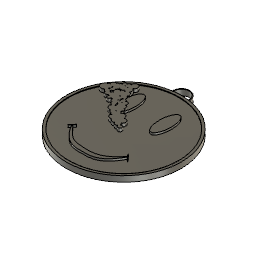
Comedian_Badge_v.2 (Autodesk Fusion 360 design; units mm, degrees)
part number: 2026-01-01-18-05-26-617
part number: 2026-01-01-18-09-21-540
part number: 2026-01-01-18-09-43-519
part number: 2026-01-01-18-09-54-607
Autodesk Fusion 360 part; units mm, degrees
sketch "Base" plane through (0, 0, 0) normal (0, 0, 1) x (1, 0, 0) in component "Base"
  circle A0 centre (0, 0) radius 32.5
  circle A1 centre (0, 0) radius 34
  arc A2 (4.9865, 33.6324) -> (-4.9865, 33.6324) centre (0, 34) ccw
  arc A3 (4.4878, 33.6691) -> (-4.4878, 33.6691) centre (0, 34) ccw
  dimension "d1" = 65
  dimension "d2" = 1.5
  dimension "d7" = 10
  dimension "d8" = -0.5
  constraint coincident A0.centre A1.centre
  constraint coincident A1 A2.centre
  constraint vertical A0.centre A2.centre
  constraint coincident A1 A2.start
  constraint coincident A1 A2.end
  measures "d1" diameter of A0
  measures "d7" diameter of A2
extrude "Face" add sketch "Base" along normal blind 3 contours A0 makes body 1 in component "Base"
extrude "Boundary" add sketch "Base" along normal blind 3.4 contours A1 bodies 1 in component "Base"
extrude "Extrude3" add sketch "Base" along normal blind 3.4 contours A1 A2 A3 bodies 1 in component "Base"
sketch "Face" plane through (0, 0, 3) normal (0, 0, 1) x (-1, 0, 0) in component "Eyes, Mouth"
  circle A0 centre (0, 0) radius 32.5
  line L0 (0, -32.5) -> (0, 32.5) construction
  line L1 (32.5, 0) -> (-32.5, 0) construction
  line L2 (32.5, 0) -> (0, 0) construction
  line L3 (16.25, 0) -> (16.25, -28.1458) construction
  line L4 (0, 0) -> (-32.5, 0) construction
  line L5 (0, 0) -> (-32.5, 0) construction
  line L6 (-16.25, 0) -> (-16.25, -28.1458) construction
  line L7 (16.25, 0) -> (16.25, 28.1458) construction
  line L8 (-16.25, 0) -> (-16.25, 28.1458) construction
  line L9 (10.514, -30.7523) -> (10.5048, 0) construction
  line L10 (-10.51, 0) -> (-10.51, -30.7537) construction
  line L11 (29.33, -14) -> (-29.33, -14) construction
  ellipse E0 centre (10.509, -14) end of major axis (10.5116, -22.6) minor radius 3.5
  line L12 (10.5064, -5.4) -> (10.5116, -22.6) construction
  line L13 (7.009, -14.001) -> (14.009, -13.999) construction
  ellipse E1 centre (-10.53, -14) end of major axis (-10.5274, -22.6) minor radius 3.5
  line L14 (15.0904, 12.7622) -> (17.4096, 15.3836)
  line L15 (16.25, 14.0729) -> (-16.25, 14.0729) construction
  line L16 (-15.0938, 12.7592) -> (-17.4062, 15.3866)
  spline S0 degree 5 poles (16.25, 14.0729) (16.3, 14.0848) (16.3341, 14.1993) (16.1818, 14.6464) (15.5759, 15.7501) (14.2531, 17.6838) (12.5268, 19.7926) (10.5746, 21.7057) (8.5494, 23.1547) (6.5388, 24.0726) (4.5785, 24.5327) (2.6673, 24.6856) (0.7818, 24.6946) (-1.1097, 24.6783) (-3.031, 24.6326) (-4.9909, 24.4416) (-6.9805, 23.9504) (-8.9701, 23.0199) (-10.9061, 21.5858) (-12.7062, 19.7261) (-14.2606, 17.6936) (-15.454, 15.8206) (-16.1842, 14.4433) (-16.3813, 13.8224) (-16.0298, 14.0561) (-15.1804, 15.0207) (-13.9095, 16.4685) (-12.276, 18.1183) (-10.3075, 19.7152) (-8.0314, 21.0469) (-5.4863, 21.9624) (-2.7594, 22.4114) (0.0273, 22.4249) (2.6134, 22.2412) (4.8105, 22.0395) (6.6671, 21.7352) (8.3079, 21.1812) (9.891, 20.2249) (11.5227, 18.8139) (13.1704, 17.1114) (14.6738, 15.4616) (15.5937, 14.498) (16.0342, 14.1281) (16.2, 14.0611) (16.25, 14.0729) knots 0 0 0 0 0 0 0.025 0.05 0.075 0.1 0.125 0.15 0.175 0.2 0.225 0.25 0.275 0.3 0.325 0.35 0.375 0.4 0.425 0.45 0.475 0.5 0.525 0.55 0.575 0.6 0.625 0.65 0.675 0.7 0.725 0.75 0.775 0.8 0.825 0.85 0.875 0.9 0.925 0.95 0.975 1 1 1 1 1 1
  line L17 (-4.0312, 22.4795) -> (4.0312, 22.2695)
  line L18 (15.3272, 12.5528) -> (17.6464, 15.1741)
  spline S1 degree 5 poles (17.6464, 15.1741) (17.6631, 15.193) (17.6879, 15.2308) (17.6992, 15.2873) (17.6702, 15.3599) (17.5911, 15.4298) (17.5155, 15.4498) (17.4608, 15.4318) (17.4263, 15.4025) (17.4096, 15.3836) knots 0 0 0 0 0 0 0.2 0.4 0.6 0.8 1 1 1 1 1 1
  spline S2 degree 5 poles (15.3272, 12.5528) (15.3104, 12.5338) (15.276, 12.5046) (15.2212, 12.4866) (15.1457, 12.5065) (15.0666, 12.5765) (15.0376, 12.649) (15.0488, 12.7055) (15.0737, 12.7433) (15.0904, 12.7622) knots 0 0 0 0 0 0 0.2 0.4 0.6 0.8 1 1 1 1 1 1
  line L19 (-15.3311, 12.5505) -> (-17.6434, 15.1778)
  spline S3 degree 5 poles (-15.3311, 12.5505) (-15.3144, 12.5315) (-15.28, 12.5022) (-15.2253, 12.484) (-15.1498, 12.5037) (-15.0705, 12.5735) (-15.0414, 12.6459) (-15.0524, 12.7024) (-15.0771, 12.7403) (-15.0938, 12.7592) knots 0 0 0 0 0 0 0.2 0.4 0.6 0.8 1 1 1 1 1 1
  spline S4 degree 5 poles (-17.4062, 15.3866) (-17.4229, 15.4056) (-17.4572, 15.4349) (-17.5119, 15.4531) (-17.5874, 15.4333) (-17.6667, 15.3636) (-17.6959, 15.2912) (-17.6848, 15.2346) (-17.6601, 15.1968) (-17.6434, 15.1778) knots 0 0 0 0 0 0 0.2 0.4 0.6 0.8 1 1 1 1 1 1
  point P0 (32.5, 0)
  point P1 (16.25, 0)
  point P2 (10.5048, 0)
  point P3 (16.25, 14.0729)
  point P4 (-16.25, 14.0729)
  point P5 (10.4983, 21.6396)
  point P6 (0, 24.6844)
  point P7 (-10.4358, 21.8495)
  point P8 (-14.4255, 15.8649)
  point P9 (0, 22.3745)
  point P10 (10.5048, 19.6447)
  dimension "d11" = 32.5
  dimension "d12" = 32.5
  dimension "d14" = 30.7523
  dimension "d15" = 5.74
  dimension "d16" = 7
  dimension "d17" = 14
  dimension "d18" = 5.4
  dimension "d23" = 30.7523
  dimension "d26" = -21.039
  dimension "d27" = 0
  dimension "d32" = 3.5
  dimension "d37" = 3.5
  dimension "d38" = 10.51
  dimension "d39" = 18.8
  dimension "d40" = 0.3161
  dimension "d42" = -0.316
  constraint coincident A0 L0.start
  constraint coincident A0 L0.end
  constraint vertical L0
  constraint coincident P0 L1.start
  constraint coincident A0 L1.end
  constraint coincident A0.centre L2.end
  constraint midpoint L2 P1
  constraint coincident A0 L3.end
  constraint perpendicular L2 L3
  constraint midpoint L4 L6.start
  constraint coincident A0 L6.end
  constraint perpendicular L5 L6
  constraint coincident A0 L7.end
  constraint parallel L3 L7
  constraint coincident A0 L8.end
  constraint perpendicular L1 L8
  constraint coincident A0 L9.start
  constraint coincident L2 P2
  constraint coincident P1 L3.start
  constraint coincident P2 L9.end
  constraint coincident A0 L10.end
  constraint coincident A0 L11.start
  constraint coincident A0 L11.end
  constraint perpendicular L6 L11
  constraint coincident E0 L12.start
  constraint coincident E0 L12.end
  constraint coincident E0 L13.start
  constraint coincident E0 L13.end
  constraint coincident L11 E0.centre
  constraint coincident L9 E0.centre
  constraint parallel L9 L12
  constraint midpoint L7 P3
  constraint coincident P3 L15.start
  constraint midpoint L8 P4
  constraint coincident P4 L15.end
  constraint coincident P3 L14
  constraint coincident P4 L16
  constraint midpoint P3 L14
  constraint midpoint P4 L16
  constraint coincident L0 P6
  constraint coincident L0 P9
  constraint midpoint P9 L17
  measures "d11" distance of A0 L0
  measures "d12" distance of L0.start L1
  measures "d14" distance of L9.start P2
  measures "d15" distance of L6.start L10.start
  measures "d17" vertical distance of P0 L11.start
  measures "d18" distance of L2 L12.start
  measures "d23" vertical distance of L9.start P2
  measures "d32" distance of L14.start L14.end
  measures "d37" distance of L16.start L16.end
  measures "d38" distance of L0 L10
  measures "d39" distance of L11.end E1.centre
extrude "Extrude1" add sketch "Face" along normal blind 1.21 separate body contours E0 | E1 | L14 S0 L18 S1 S2 | L14 L16 S0 | L16 S0 L19 S3 S4 makes body 2 at (-9.4455, 16.4516, 3) makes body 3 at (11.5935, 16.4516, 3) makes body 4 at (-16.1002, -13.4265, 3.4033) in component "Eyes, Mouth"
sketch "Splatter " plane through (0, 0, 3) normal (0, 0, 1) x (-1, 0, 0) in component "Blood Splatter"
  circle A0 centre (0, 0) radius 32.5
  ellipse E0 centre (10.509, -14) end of major axis (10.5116, -22.6) minor radius 3.5
  arc A1 (25.4629, -17.5215) -> (26.3142, -16.9273) centre (24.9293, -15.8501) ccw
  arc A2 (23.5835, -16.9759) -> (23.4741, -17.039) centre (24.2368, -18.2353) ccw
  arc A3 (23.7521, -19.5687) -> (25.4629, -17.5215) centre (24.2368, -18.2353) ccw
  arc A4 (23.4741, -17.039) -> (22.9658, -16.2432) centre (21.9285, -17.4659) ccw
  arc A5 (23.6662, -14.6323) -> (23.2521, -15.3347) centre (24.9293, -15.8501) ccw
  arc A6 (23.1755, -15.9018) -> (23.5835, -16.9759) centre (24.9293, -15.8501) ccw
  arc A7 (22.9658, -16.2432) -> (23.1755, -15.9018) centre (22.0824, -15.4654) ccw
  arc A8 (23.0153, -14.7478) -> (23.6657, -14.6525) centre (23.1596, -13.4649) ccw
  arc A9 (22.6208, -20.2196) -> (23.7521, -19.5687) centre (22.8518, -19.3125) ccw
  arc A10 (21.9285, -20.8465) -> (22.6208, -20.2196) centre (22.0055, -20.2358) ccw
  arc A11 (21.861, -21.1496) -> (21.9285, -20.8465) centre (21.236, -20.8513) ccw
  arc A12 (20.3783, -22.3478) -> (21.861, -21.1496) centre (20.869, -21.4386) ccw
  arc A13 (18.7605, -23.1553) -> (20.3783, -22.3478) centre (19.1586, -21.9285) ccw
  arc A14 (16.2635, -21.6655) -> (18.7605, -23.1553) centre (16.9273, -23.3904) ccw
  arc A15 (18.5437, -20.8482) -> (18.5837, -20.7739) centre (16.9273, -19.928) ccw
  arc A16 (18.4968, -20.8215) -> (18.5437, -20.8482) centre (19.3894, -19.3125) ccw
  arc A17 (20.004, -20.9544) -> (19.9713, -20.927) centre (19.1586, -21.9285) ccw
  arc A18 (18.5837, -20.7739) -> (18.4968, -20.8215) centre (19.1586, -21.9285) ccw
  arc A19 (19.9713, -20.927) -> (19.9456, -20.9751) centre (20.869, -21.4386) ccw
  arc A20 (19.9456, -20.9751) -> (20.004, -20.9544) centre (19.3894, -19.3125) ccw
  arc A21 (17.9205, -18.3555) -> (17.2298, -18.0929) centre (16.9273, -19.928) ccw
  arc A22 (15.4231, -18.8341) -> (16.2635, -21.6655) centre (16.9273, -19.928) ccw
  arc A23 (14.0027, -16.0094) -> (15.4231, -18.8341) centre (15.6962, -16.9273) ccw
  arc A24 (13.0581, -14.0375) -> (14.0027, -16.0094) centre (14.696, -14.4651) ccw
  arc A25 (11.9128, -13.0213) -> (13.0581, -14.0375) centre (13.1571, -12.7724) ccw
  arc A26 (10.0097, -11.0551) -> (11.9128, -13.0213) centre (11.1566, -11.8491) ccw
  arc A27 (14.007, -13.7147) -> (13.8846, -11.7327) centre (13.1571, -12.7724) ccw
  arc A28 (12.5392, -11.664) -> (12.4165, -11.2504) centre (11.1566, -11.8491) ccw
  arc A29 (12.4448, -11.3402) -> (12.454, -11.3366) centre (11.926, -10.0025) ccw
  arc A30 (12.4448, -11.3402) -> (12.5006, -11.4757) centre (13.7688, -10.8739) ccw
  arc A31 (8.5906, -8.9041) -> (10.0097, -11.0551) centre (9.8486, -9.6178) ccw
  arc A32 (12.0159, -8.5705) -> (12.2514, -7.9548) centre (10.8489, -7.7712) ccw
  arc A33 (12.7723, -8.0051) -> (13.0075, -7.9812) centre (12.6955, -6.0784) ccw
  arc A34 (21.0905, -16.0989) -> (20.375, -17.8625) centre (21.9285, -17.4659) ccw
  arc A35 (21.0725, -18.8216) -> (22.3889, -19.0017) centre (21.9285, -17.4659) ccw
  arc A36 (20.5978, -20.5828) -> (21.0725, -18.8216) centre (19.3894, -19.3125) ccw
  arc A37 (20.375, -17.8625) -> (17.9205, -18.3555) centre (19.3894, -19.3125) ccw
  arc A38 (20.3616, -14.1581) -> (20.9744, -13.3668) centre (19.3894, -12.7724) ccw
  arc A39 (24.3803, -13.0447) -> (23.1072, -12.175) centre (23.1596, -13.4649) ccw
  arc A40 (21.8718, -13.5557) -> (22.168, -14.2915) centre (23.1596, -13.4649) ccw
  arc A41 (20.9744, -13.3668) -> (21.8718, -13.5557) centre (21.6977, -12.1569) ccw
  arc A42 (23.1072, -12.175) -> (20.468, -11.4678) centre (21.6977, -12.1569) ccw
  arc A43 (23.2521, -15.3347) -> (23.0153, -14.7478) centre (22.0824, -15.4654) ccw
  arc A44 (23.6662, -14.6323) -> (23.6657, -14.6525) centre (25.9295, -14.696) ccw
  arc A45 (26.3142, -16.9273) -> (24.3803, -13.0447) centre (25.9295, -14.696) ccw
  arc A46 (20.3275, -17.3792) -> (20.0415, -17.6851) centre (21.1591, -18.4434) ccw
  arc A47 (10.7877, -6.3579) -> (10.608, -6.3773) centre (10.8489, -7.7712) ccw
  arc A48 (20.468, -11.4678) -> (19.8146, -11.134) centre (19.3894, -12.7724) ccw
  arc A49 (17.7423, -13.1625) -> (17.7591, -13.2277) centre (19.3894, -12.7724) ccw
  arc A50 (18.7501, -11.459) -> (18.6635, -11.2432) centre (17.4659, -11.8491) ccw
  arc A51 (19.8146, -11.134) -> (18.7501, -11.459) centre (19.0047, -10.3872) ccw
  arc A52 (1.8883, 1.6496) -> (1.4604, 0.6155) centre (0.6925, 1.5388) ccw
  arc A53 (4.3266, 1.0325) -> (1.8883, 1.6496) centre (2.9238, 0.6155) ccw
  arc A54 (1.4604, 0.6155) -> (2.0753, -0.5768) centre (2.9238, 0.6155) ccw
  arc A55 (7.09, -0.027) -> (4.3266, 1.0325) centre (5.309, -0.5386) ccw
  arc A56 (6.4152, -1.7823) -> (6.4771, -1.9771) centre (8.002, -1.385) ccw
  arc A57 (9.3855, -2.2578) -> (7.09, -0.027) centre (8.002, -1.385) ccw
  arc A58 (12.65, -8.7637) -> (12.0159, -8.5705) centre (11.926, -10.0025) ccw
  arc A59 (14.1794, -10.1318) -> (15.6627, -8.7834) centre (15.6962, -10.3103) ccw
  arc A60 (12.9133, -7.7539) -> (14.1794, -10.1318) centre (14.1574, -8.6175) ccw
  arc A61 (15.6627, -8.7834) -> (14.3231, -7.1122) centre (14.1574, -8.6175) ccw
  arc A62 (2.0753, -0.5768) -> (3.5349, -3.9874) centre (2.9238, -2.2313) ccw
  arc A63 (10.7291, -3.0846) -> (9.3855, -2.2578) centre (9.6178, -3.3855) ccw
  arc A64 (9.9419, -5.5128) -> (10.1672, -5.6716) centre (10.8489, -4.4651) ccw
  arc A65 (10.2023, -5.5388) -> (9.9996, -5.5601) centre (10.1564, -6.0784) ccw
  arc A66 (10.6401, -5.835) -> (10.781, -5.8492) centre (10.8489, -4.4651) ccw
  arc A67 (12.2113, -4.212) -> (10.7291, -3.0846) centre (10.8489, -4.4651) ccw
  arc A68 (14.3231, -7.1122) -> (12.2113, -4.212) centre (12.6955, -6.0784) ccw
  arc A69 (8.2363, -6.5941) -> (8.5906, -8.9041) centre (8.7714, -7.6942) ccw
  arc A70 (7.3368, -5.5208) -> (7.4363, -5.8313) centre (8.7714, -5.2321) ccw
  arc A71 (3.5349, -3.9874) -> (6.628, -5.9898) centre (5.7707, -3.9241) ccw
  arc A72 (6.9972, -5.7944) -> (7.3368, -5.5208) centre (5.7707, -3.9241) ccw
  arc A73 (7.4363, -5.8313) -> (6.9972, -5.7944) centre (7.1556, -6.5401) ccw
  arc A74 (6.628, -5.9898) -> (7.9073, -6.4131) centre (7.1556, -6.5401) ccw
  arc A75 (16.9585, -15.4723) -> (17.7624, -15.5478) centre (17.4659, -14.3882) ccw
  arc A76 (16.4914, -14.0679) -> (16.2814, -14.2163) centre (17.1581, -15.2346) ccw
  arc A77 (17.3988, -17.8282) -> (18.9065, -17.0212) centre (17.9275, -17.0042) ccw
  arc A78 (17.2298, -18.0929) -> (17.3988, -17.8282) centre (15.6962, -16.9273) ccw
  arc A79 (17.4568, -16.1458) -> (16.9585, -15.4723) centre (15.6962, -16.9273) ccw
  arc A80 (16.2913, -14.1578) -> (16.4914, -14.0679) centre (15.927, -13.0802) ccw
  arc A81 (17.0493, -13.2661) -> (17.0635, -13.1295) centre (15.927, -13.0802) ccw
  arc A82 (16.3598, -14.1537) -> (16.3281, -14.0164) centre (14.696, -14.4651) ccw
  arc A83 (14.945, -11.64) -> (14.9806, -11.5823) centre (13.7688, -10.8739) ccw
  arc A84 (15.7541, -11.9558) -> (15.6784, -11.8374) centre (15.1226, -12.2758) ccw
  arc A85 (14.9806, -11.5823) -> (14.8899, -11.6073) centre (15.1226, -12.2758) ccw
  arc A86 (17.9213, -10.5866) -> (17.2073, -10.5321) centre (17.4659, -11.8491) ccw
  arc A87 (16.1257, -11.7759) -> (16.1284, -11.9606) centre (17.4659, -11.8491) ccw
  arc A88 (17.7591, -13.2277) -> (17.4659, -13.1913) centre (17.4659, -14.3882) ccw
  arc A89 (16.3281, -14.0164) -> (16.2814, -14.2163) centre (17.4659, -14.3882) ccw
  arc A90 (18.9065, -17.0212) -> (20.9715, -15.8541) centre (19.3894, -15.4654) ccw
  arc A91 (20.9715, -15.0766) -> (20.3616, -14.1581) centre (19.3894, -15.4654) ccw
  arc A92 (22.168, -14.2915) -> (20.9715, -15.0766) centre (22.0824, -15.4654) ccw
  arc A93 (20.9715, -15.8541) -> (21.0905, -16.0989) centre (22.0824, -15.4654) ccw
  arc A94 (7.9073, -6.4131) -> (8.2363, -6.5941) centre (8.7714, -5.2321) ccw
  arc A95 (10.1672, -5.6716) -> (10.2215, -5.4286) centre (8.7714, -5.2321) ccw
  constraint tangent A4 A90
  constraint coincident A1.end A44
  constraint concentric A1 A5
  constraint concentric A2 A3
  constraint coincident A46.start A4
  constraint coincident A34.start A4
  constraint concentric A4 A34
  constraint coincident A5.end A7
  constraint concentric A5 A6
  constraint concentric A7 A43
  constraint coincident A40.end A43
  constraint concentric A8 A39
  constraint coincident A36.start A16
  constraint coincident A19.end A16
  constraint coincident A17.start A16
  constraint concentric A13 A17
  constraint coincident A21.start A15
  constraint coincident A15.end A17
  constraint concentric A15 A21
  constraint concentric A16 A20
  constraint concentric A17 A18
  constraint concentric A20 A36
  constraint concentric A21 A22
  constraint concentric A23 A78
  constraint coincident E0 A27.start
  constraint coincident A25.start A27
  constraint concentric A25 A27
  constraint concentric A26 A28
  constraint coincident E0 A27.end
  constraint coincident A28 A29.end
  constraint concentric A32 A47
  constraint coincident A33.start A60
  constraint coincident E0 A33.end
  constraint concentric A33 A68
  constraint coincident E0 A60.start
  constraint coincident A34.end A36
  constraint concentric A34 A35
  constraint concentric A36 A37
  constraint coincident A75.end A90
  constraint coincident A49.end A38
  constraint concentric A38 A48
  constraint coincident A39.end A41
  constraint concentric A39 A40
  constraint concentric A41 A42
  constraint concentric A43 A92
  constraint concentric A44 A45
  constraint coincident A37 A46.end
  constraint coincident A49.start A48
  constraint concentric A48 A49
  constraint coincident A86.start A51
  constraint concentric A50 A86
  constraint concentric A53 A54
  constraint concentric A56 A57
  constraint coincident A58.start A60
  constraint coincident A83.end A84
  constraint coincident A59.end A60
  constraint concentric A60 A61
  constraint coincident A65.end A64
  constraint coincident E0 A64.start
  constraint coincident A64.end A70
  constraint concentric A64 A66
  constraint coincident A65.start A70
  constraint coincident A66.end A68
  constraint concentric A66 A67
  constraint coincident A69.start A70
  constraint coincident A74.end A70
  constraint concentric A70 A94
  constraint coincident A71.end A73
  constraint concentric A71 A72
  constraint concentric A73 A74
  constraint coincident A75.start A88
  constraint concentric A75 A88
  constraint coincident A76 A82.start
  constraint coincident A79.start A78
  constraint concentric A78 A79
  constraint coincident A80.start A88
  constraint coincident A81.start A88
  constraint concentric A80 A81
  constraint coincident A82.end A88
  constraint coincident A59 A83.start
  constraint coincident A59 A85.end
  constraint coincident A59 A84.end
  constraint concentric A84 A85
  constraint coincident A59 A86.end
  constraint coincident A59 A87.start
  constraint concentric A86 A87
  constraint coincident A28 A30.end
  constraint concentric A88 A89
  constraint coincident A90.end A92
  constraint concentric A90 A91
  constraint concentric A92 A93
  constraint concentric A94 A95
extrude "Extrude5" add sketch "Splatter " along normal blind 1.9359 and the other way up to surface (0 mm away) separate body contours E0 A24 A25 A26 A31 A60 A64 A69 A95 | E0 A1 A3 A9 A10 A11 A12 A13 A14 A22 A23 A24 A27 A39 A42 A45 A48 A51 A59 A60 A86 | E0 A52 A53 A54 A55 A57 A59 A60 A61 A62 A63 A67 A68 A69 A71 A74 A83 A85 makes body 5 in component "Blood Splatter"
extrude "Extrude4" [suppressed] in component "Blood Splatter"
fillet "Fillet2" [suppressed] in component "Base"
extrude "Extrude2" [suppressed] in component "Blood Splatter"
extrude "Extrude3'" [suppressed] in component "Blood Splatter"
fillet "Fillet1" [suppressed] in component "Base"
component "Base" placed x (1, 0, 0) y (0, 1, 0) z (0, 0, 1) at (0, 0, 0)
component "Eyes, Mouth" placed x (1, 0, 0) y (0, 1, 0) z (0, 0, 1) at (0, 0, 0)
component "Blood Splatter" placed x (1, 0, 0) y (0, 1, 0) z (0, 0, 1) at (0, 0, 0)
named bodies: "Base", "Left Eye", "Right Eye", "Mouth", "Splatter"
